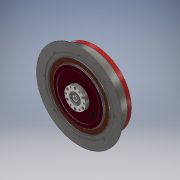
# Autodesk Inventor part: Motor Mitsuba M2096 D-III
Saved by Autodesk Inventor 2018 (Build 220112000, 112)
## iProperties
Created: 2017-11-30
Part Number: Motor Mitsuba M2096 D-III
Material: Stainless Steel
Document SubType Name: Modeling
Designer: Albert Theodore
Density: 8 g/cm^3
Appearance: Semi-Polished
Author: Albert Theodore
Autodesk Inventor part; units mm, degrees
ref_plane "XZ Plane" through (0, 0, 0) normal (0, 1, 0) x (-1, 0, 0)
ref_plane "XY Plane" through (0, 0, 0) normal (0, 0, 1) x (1, 0, 0)
sketch "Sketch1" plane through (0, 0, 0) normal (0, 1, 0) x (-1, 0, 0)
  circle A0 centre (0, 0) radius 131
  dimension "d0" = 262
  constraints: 1 centre point, 1 coincident
  measures "d0" diameter of A0
extrude "Extrusion1" add sketch "Sketch1" along normal blind 14
sketch "Sketch2" plane through (0, 0, 0) normal (0, -1, 0) x (1, 0, 0)
  circle A0 centre (0, 0) radius 130.5
  dimension "d3" = 261
  constraints: 1 centre point, 1 coincident
  measures "d3" diameter of A0
extrude "Extrusion2" add sketch "Sketch2" along normal blind 42
sketch "Sketch3" plane through (0, 14, 0) normal (0, 1, 0) x (1, 0, 0)
  circle A0 centre (0, 0) radius 47
  dimension "d6" = 94
  constraints: 1 centre point, 1 coincident
  measures "d6" diameter of A0
extrude "Extrusion3" add sketch "Sketch3" along normal blind 21.5
sketch "Sketch4" plane through (0, 35.5, 0) normal (0, 1, 0) x (1, 0, 0)
  circle A0 centre (0, 0) radius 36.5
  dimension "d9" = 73
  constraints: 1 centre point, 1 coincident
  measures "d9" diameter of A0
extrude "Extrusion4" add sketch "Sketch4" along normal blind 13.5
thread "Thread1" size "M75x1.5" class "6g" standard "ANSI Metric M Profile" full length
sketch "Sketch5" plane through (0, 14, 0) normal (0, 1, 0) x (1, 0, 0)
  circle A0 centre (0, 0) radius 58
  line L0 (4, -54) -> (-4, -54)
  line L1 (-4, -54) -> (4, -54)
  line L2 (8, -57.4456) -> (8, -58)
  line L3 (4, -62) -> (-4, -62)
  line L4 (-8, -58) -> (-8, -57.4456)
  arc A1 (-4, -54) -> (-4, -62) centre (-4, -58) ccw
  arc A2 (4, -62) -> (4, -54) centre (4, -58) ccw
  arc A3 (51.6936, 34.4641) -> (44.7654, 30.4641) centre (48.2295, 32.4641) ccw
  line L5 (51.6936, 34.4641) -> (55.6936, 27.5359)
  arc A4 (48.7654, 23.5359) -> (55.6936, 27.5359) centre (52.2295, 25.5359) ccw
  line L6 (44.7654, 30.4641) -> (48.7654, 23.5359)
  arc A5 (-55.6936, 27.5359) -> (-48.7654, 23.5359) centre (-52.2295, 25.5359) ccw
  line L7 (-55.6936, 27.5359) -> (-51.6936, 34.4641)
  arc A6 (-44.7654, 30.4641) -> (-51.6936, 34.4641) centre (-48.2295, 32.4641) ccw
  line L8 (-48.7654, 23.5359) -> (-44.7654, 30.4641)
  circle A7 centre (-58, 0) radius 4
  circle A8 centre (0, 0) radius 58
  circle A9 centre (-29, -50.2295) radius 4
  circle A10 centre (29, -50.2295) radius 4
  circle A11 centre (58, 0) radius 4
  circle A12 centre (29, 50.2295) radius 4
  circle A13 centre (-29, 50.2295) radius 4
  point P0 (46.2295, 35.9282)
  point P1 (54.2295, 22.0718)
  point P2 (-54.2295, 22.0718)
  point P3 (-46.2295, 35.9282)
  dimension "d16" = 116
  dimension "d18" = 8
  dimension "d21" = 8
  dimension "d24" = 360
  dimension "d28" = 8
  dimension "d31" = 360
  constraints: 21 point on circle, 18 end point, 14 centre point, 3 tangent, 2 coincident, 2 perpendicular, 1 concentric, 1 horizontal, 1 vertical, 50 other
  measures "d16" diameter of A0
  measures "d18" distance of L0.start L0.end
  measures "d21" diameter of A1
  measures "d28" diameter of A7
extrude "Extrusion5" add sketch "Sketch5" along normal blind 4 contours A4 L6 A3 A0 | A0 A3 L5 A4 | A2 L3 A1 A0 | A0 A1 L0 A2 | A6 L8 A5 A0 | A0 A5 L7 A6
extrude "Extrusion6" cut sketch "Sketch5" against normal blind 10 contours A0 A11 | A0 A11 | A10 A0 | A0 A10 | A12 A0 | A0 A12 | A13 A0 | A0 A13 | A9 A0 | A0 A9 | A7 A0 | A0 A7
sketch "Sketch6" plane through (0, 14, 0) normal (0, 1, 0) x (1, 0, 0)
  circle A0 centre (0, -127.5) radius 3
  circle A1 centre (0, 0) radius 127.5
  circle A2 centre (90.1561, -90.1561) radius 3
  circle A3 centre (127.5, 0) radius 3
  circle A4 centre (90.1561, 90.1561) radius 3
  circle A5 centre (0, 127.5) radius 3
  circle A6 centre (-90.1561, 90.1561) radius 3
  circle A7 centre (-127.5, 0) radius 3
  circle A8 centre (-90.1561, -90.1561) radius 3
  dimension "d35" = 6
  dimension "d36" = 127.5
  dimension "d39" = 360
  constraints: 8 centre point, 1 coincident, 1 vertical alignment, 19 other
  measures "d35" diameter of A0
  measures "d36" distance of point (0, 0) A0.centre
hole "Hole1" at (0, 14, 127.5) direction (0, -1, 0) diameter 3 depth 8 tip angle 118 counterbore diameter 6 counterbore depth 2
pattern_circular "Circular Pattern1" count 8 over 360 about axis through (0, 0, 0) along (0, 1, 0) of "Hole1"
sketch "Sketch7" plane through (0, -42, 0) normal (0, -1, 0) x (1, 0, 0)
  circle A0 centre (0, 0) radius 38.5
  dimension "d51" = 77
  constraints: 1 centre point, 1 coincident
  measures "d51" diameter of A0
extrude "Extrusion7" add sketch "Sketch7" along normal blind 17
sketch "Sketch8" plane through (0, -42, 0) normal (0, -1, 0) x (1, 0, 0)
  circle A0 centre (0, 0) radius 90
  dimension "d54" = 180
  constraints: 1 centre point, 1 coincident
  measures "d54" diameter of A0
extrude "Extrusion8" add sketch "Sketch8" along normal blind 4
ref_plane "Work Plane1" through (0, 0, 0) normal (1, 0, 0) x (0, 1, 0)
sketch "Sketch9" plane through (0, 0, 0) normal (1, 0, 0) x (0, 1, 0)
  line L0 (-42, 130.5) -> (-42, -130.5) projected
  line L1 (-42, 93.7788) -> (-43, 93.7788)
  line L2 (-43, 93.7788) -> (-43, 92.7788)
  line L3 (-43, 92.7788) -> (-46, 92.7788)
  line L4 (-46, 92.7788) -> (-46, 91.2788)
  line L5 (-46, 91.2788) -> (-42, 91.2788)
  line L6 (-42, 93.7788) -> (-42, 91.2788)
  line L7 (-42, 108.7788) -> (-43, 108.7788)
  line L8 (-43, 108.7788) -> (-43, 109.7788)
  line L9 (-43, 109.7788) -> (-46, 109.7788)
  line L10 (-46, 109.7788) -> (-46, 111.2788)
  line L11 (-46, 111.2788) -> (-42, 111.2788)
  line L12 (-42, 111.2788) -> (-42, 108.7788)
  line L13 (62.3394, 0) -> (-88.5963, 0)
  point P0 (0, 0)
  dimension "d58" = 1
  dimension "d59" = 1
  dimension "d60" = 1.5
  dimension "d61" = 4
  dimension "d62" = 15
  dimension "d63" = 1
  dimension "d64" = 1.5
  constraints: 26 end point, 9 perpendicular, 4 point on line, 3 horizontal, 1 parallel
  measures "d58" distance between parallel lines of L0 L2
  measures "d59" distance between parallel lines of L1 L3
  measures "d60" distance of L3.end L4.end
  measures "d61" distance between parallel lines of L0 L4
  measures "d62" distance between parallel lines of L1 L7
  measures "d63" distance of L7.end L8.end
  measures "d64" distance of L9.end L10.end
revolve "Revolution1" add sketch "Sketch9" angle 360 about axis through (0, 62.3394, 0) along (0, -1, 0)
sketch "Sketch10" plane through (0, 49, 0) normal (0, 1, 0) x (1, 0, 0)
  circle A0 centre (0, 0) radius 32.5
  dimension "d66" = 65
  constraints: 1 centre point, 1 coincident
  measures "d66" diameter of A0
extrude "Extrusion9" cut sketch "Sketch10" against normal blind 20
chamfer "Chamfer1" distance 2 angle 45 1 edges at (-36.5, 49, 0)
sketch "Sketch11" plane through (0, 0, 0) normal (1, 0, 0) x (0, 1, 0)
  line L0 (-42, 155) -> (-44, 155)
  line L1 (0, 0) -> (-90.776, 0)
  line L2 (-42, 124) -> (-44, 124)
  line L3 (-44, 155) -> (-44, 124)
  line L4 (-42, 155) -> (-42, 124)
  line L5 (-42, 130.5) -> (-42, -130.5) projected
  dimension "d72" = 2
  dimension "d73" = 155
  dimension "d74" = 124
  constraints: 10 end point, 3 horizontal, 1 collinear, 1 vertical
  measures "d72" distance of L0.start L0.end
  measures "d73" distance between parallel lines of L1 L0
  measures "d74" distance between parallel lines of L1 L2
revolve "Revolution2" add sketch "Sketch11" angle 360 about axis through (0, 0, 0) along (0, -1, 0)
sketch "Sketch12" plane through (0, -44, 0) normal (0, -1, 0) x (1, 0, 0)
  circle A0 centre (0, 127.5) radius 3 projected
  point P0 (0, 0)
hole "Hole2" at (0, -44, 127.5) direction (0, 1, 0) diameter 3 depth 8 tip angle 118 counterbore diameter 6 counterbore depth 2
pattern_circular "Circular Pattern2" count 8 over 360 about axis through (0, 0, 0) along (0, -1, 0) of "Hole2"
sketch "Sketch13" plane through (0, -59, 0) normal (0, -1, 0) x (1, 0, 0)
  circle A0 centre (0, 0) radius 32
  circle A1 centre (0, 32) radius 4
  dimension "d86" = 64
  dimension "d87" = 8
  constraints: 1 centre point, 1 coincident, 1 vertical alignment, 2 other
  measures "d87" diameter of A1
hole "Hole3" at (0, -59, 32) direction (0, 1, 0) diameter 8 depth 8
thread "Thread2" size "M8x1.25" class "6H" standard "ANSI Metric M Profile" full length
pattern_circular "Circular Pattern3" count 6 over 360 about axis through (0, -42, 0) along (0, -1, 0) of "Hole3"
sketch "Sketch14" plane through (0, -59, 0) normal (0, -1, 0) x (1, 0, 0)
  circle A0 centre (0, 0) radius 32
  circle A1 centre (32, 0) radius 2.5
  dimension "d100" = 64
  dimension "d101" = 5
  constraints: 1 centre point, 1 coincident, 1 horizontal alignment, 2 other
  measures "d101" diameter of A1
hole "Hole4" at (32, -59, 0) direction (0, 1, 0) diameter 5 depth 8
pattern_circular "Circular Pattern4" count 6 over 360 about axis through (0, 48, 0) along (0, 1, 0) of "Hole4"
thread "Thread3" size "M8x1.25" class "6H" standard "ANSI Metric M Profile" full length
thread "Thread4" size "M8x1.25" class "6H" standard "ANSI Metric M Profile" full length
thread "Thread5" size "M8x1.25" class "6H" standard "ANSI Metric M Profile" full length
thread "Thread6" size "M8x1.25" class "6H" standard "ANSI Metric M Profile" full length
thread "Thread7" size "M8x1.25" class "6H" standard "ANSI Metric M Profile" full length
thread "Thread8" size "M5x0.8" class "6H" standard "ANSI Metric M Profile" full length
thread "Thread9" size "M5x0.8" class "6H" standard "ANSI Metric M Profile" full length
thread "Thread10" size "M5x0.8" class "6H" standard "ANSI Metric M Profile" full length
thread "Thread11" size "M5x0.8" class "6H" standard "ANSI Metric M Profile" full length
thread "Thread12" size "M5x0.8" class "6H" standard "ANSI Metric M Profile" full length
thread "Thread13" size "M5x0.8" class "6H" standard "ANSI Metric M Profile" full length
sketch "Sketch15" plane through (0, -59, 0) normal (0, -1, 0) x (1, 0, 0)
  circle A0 centre (0, 0) radius 20
  circle A1 centre (0, 0) radius 47 projected
  circle A2 centre (0, 0) radius 10
  circle A3 centre (0, 0) radius 5
  dimension "d134" = 40
  dimension "d135" = 20
  dimension "d136" = 10
  constraints: 3 centre point, 3 coincident
  measures "d134" diameter of A0
  measures "d135" diameter of A2
  measures "d136" diameter of A3
extrude "Extrusion10" cut sketch "Sketch15" against normal blind 5 contours A0 | A3
sketch "Sketch16" plane through (0, -46, 0) normal (0, -1, 0) x (1, 0, 0)
  circle A0 centre (0, 0) radius 77.5
  circle A1 centre (0, 0) radius 90 projected
  dimension "d139" = 155
  constraints: 1 centre point, 1 coincident
  measures "d139" diameter of A0
extrude "Extrusion11" add sketch "Sketch16" along normal blind 2
sketch "Sketch17" plane through (0, -46, 0) normal (0, -1, 0) x (1, 0, 0)
  circle A0 centre (51.6668, -29.8298) radius 9
  circle A1 centre (27.7128, -16) radius 4 projected
  circle A2 centre (32, 0) radius 2.5 projected
  circle A3 centre (16, -27.7128) radius 2.5 projected
  point P0 (0, 0)
  dimension "d142" = 18
  constraints: 1 centre point
  measures "d142" diameter of A0
extrude "Extrusion12" cut sketch "Sketch17" against normal blind 2 contours A0
body "Solid1"
